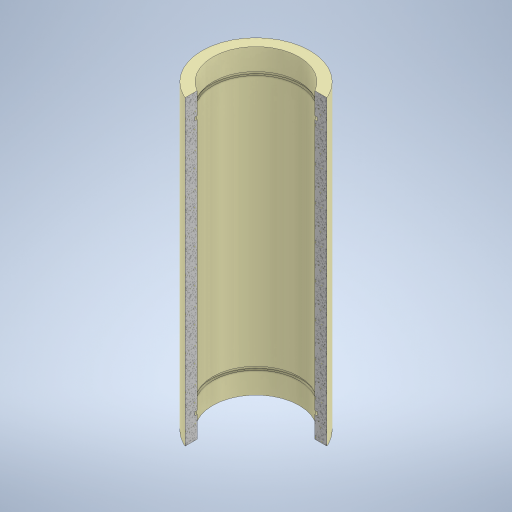
# Autodesk Inventor part: корпус
Saved by Autodesk Inventor 2024.2 (Build 282272000, 272)
## iProperties
Created: 2024-02-27
Part Number: корпус
Material: Типовые
Document SubType Name: Modeling
Designer: user
Density: 1 g/cm^3
Appearance: По умолчанию
Author: user
Autodesk Inventor part; units mm, degrees
ref_plane "YZ Plane" through (0, 0, 0) normal (1, 0, 0) x (0, 1, 0)
ref_plane "XZ Plane" through (0, 0, 0) normal (0, 1, 0) x (-1, 0, 0)
ref_plane "XY Plane" through (0, 0, 0) normal (0, 0, 1) x (1, 0, 0)
sketch "Эскиз1" plane through (0, 0, 0) normal (0, 0, 1) x (1, 0, 0)
  line L0 (0, 0) -> (0, -140)
  line L1 (0, 0) -> (20, 0) construction
  line L2 (25, 0) -> (25, -140)
  line L3 (25, -140) -> (20, -140)
  line L4 (20, 0) -> (20, -10)
  line L5 (20, -10) -> (21, -10)
  line L6 (21, -10) -> (21, -11.6)
  line L7 (21, -11.6) -> (20, -11.6)
  line L8 (20, -11.6) -> (20, -128.4)
  line L9 (20, -128.4) -> (21, -128.4)
  line L10 (21, -128.4) -> (21, -130)
  line L11 (21, -130) -> (20, -130)
  line L12 (20, -130) -> (20, -140)
  line L13 (20, -140) -> (0, -140) construction
  line L14 (20, 0) -> (25, 0)
  point P0 (20, -7)
  dimension "d0" = 140
  dimension "d1" = 50
  dimension "d3" = 42
  dimension "d4" = 40
  dimension "d5" = 1.6
  dimension "d6" = 1.6
  dimension "d13" = 10
  dimension "d14" = 10
  constraints: 30 end point, 10 perpendicular, 3 horizontal, 3 point on line, 2 collinear, 2 vertical
  measures "d0" distance of L0.start L0.end
  measures "d1" diameter of L2 L0
  measures "d3" diameter of L6 L0
  measures "d4" diameter of L4 L0
  measures "d5" distance of L5.end L6.end
  measures "d6" distance of L9.end L10.end
  measures "d13" distance between parallel lines of L5 L14
  measures "d14" distance between parallel lines of L3 L11
revolve "Вращение1" add sketch "Эскиз1" angle 360 about axis through (0, 0, 0) along (0, -1, 0)
equation "\"d14\" = my_parameter"
equation "\"my_parameter\" = 10"
